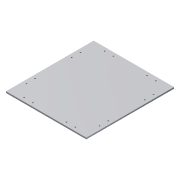
# Autodesk Inventor part: BackPlate
Saved by Autodesk Inventor 2014 (Build 180170000, 170)
## iProperties
Created: 2014-08-10
Part Number: BackPlate
Material: Generic
Document SubType Name: Modeling
Designer: Peele
Density: 1 g/cm^3
Appearance: White
Author: Peele
Autodesk Inventor part; units mm, degrees
ref_plane "YZ Plane" through (0, 0, 0) normal (1, 0, 0) x (0, 1, 0)
ref_plane "XZ Plane" through (0, 0, 0) normal (0, 1, 0) x (-1, 0, 0)
ref_plane "XY Plane" through (0, 0, 0) normal (0, 0, 1) x (1, 0, 0)
sketch "Sketch1" plane through (0, 0, 0) normal (0, 0, 1) x (1, 0, 0)
  line L0 (-112.5, -125) -> (112.5, -125)
  line L1 (112.5, -125) -> (112.5, 125)
  line L2 (112.5, 125) -> (-112.5, 125)
  line L3 (-112.5, 125) -> (-112.5, -125)
  line L4 (-112.5, -125) -> (112.5, 125) construction
  line L5 (112.5, -125) -> (-112.5, 125) construction
  point P0 (0, 0)
  dimension "d0" = 250
  dimension "d1" = 225
  constraints: 12 end point, 2 midpoint, 2 parallel, 1 horizontal, 1 perpendicular
  measures "d0" distance of L2.end L0.start
  measures "d1" distance of L1.end L2.end
extrude "Extrusion1" add sketch "Sketch1" along normal blind 5
sketch "Sketch2" plane through (0, 0, 5) normal (0, 0, 1) x (1, 0, 0)
  line L0 (112.5, -125) -> (112.5, 125) projected
  line L1 (112.5, 125) -> (-112.5, 125) projected
  line L2 (-112.5, 125) -> (-112.5, -125) projected
  circle A0 centre (-87.5, 137.5) radius 2.25
  circle A1 centre (-57.5, 137.5) radius 2.25
  circle A2 centre (57.5, 137.5) radius 2.25
  circle A3 centre (87.5, 137.5) radius 2.25
  circle A4 centre (125, 92.5) radius 2.25
  circle A5 centre (125, 62.5) radius 2.25
  circle A6 centre (-125, 92.5) radius 2.25
  circle A7 centre (-125, 62.5) radius 2.25
  line L3 (-112.5, 0) -> (-112.5, 125)
  line L4 (-112.5, 125) -> (112.5, 125)
  line L5 (112.5, 125) -> (112.5, 0)
  line L6 (112.5, 0) -> (137.5, 0)
  line L7 (137.5, 0) -> (137.5, 150)
  line L8 (137.5, 150) -> (-137.5, 150)
  line L9 (-137.5, 150) -> (-137.5, 0)
  line L10 (-137.5, 0) -> (-112.5, 0)
  point P0 (0, 0)
  dimension "d7" = 12.5
  dimension "d8" = 12.5
  dimension "d9" = 4.5
  dimension "d10" = 30
  dimension "d11" = 30
  dimension "d12" = 30
  dimension "d24" = 25
  dimension "d25" = 25
  dimension "d26" = 32.5
  dimension "d27" = 12.5
  dimension "d28" = 25
  dimension "d29" = 25
  constraints: 16 end point, 8 centre point, 7 equal radius, 5 horizontal alignment, 3 collinear, 3 perpendicular, 2 midpoint, 2 vertical alignment, 1 horizontal, 1 parallel
  measures "d7" distance from line of A0.centre L1
  measures "d8" distance from line of A6.centre L2
  measures "d9" diameter of A4
  measures "d10" distance of A3.centre A2.centre
  measures "d11" distance of A0.centre A1.centre
  measures "d12" distance of A5.centre A4.centre
  measures "d24" distance from line of A3.centre L0
  measures "d25" distance from line of A0.centre L2
  measures "d26" distance from line of A4.centre L1
  measures "d27" distance from line of A4.centre L0
  measures "d28" distance of L9.end L3.start
  measures "d29" distance between parallel lines of L8 L1
extrude "Extrusion2" add sketch "Sketch2" against normal blind 5
mirror "Mirror1" about plane through (0, 0, 0) normal (0, 1, 0) of "Extrusion2"
equation "\"d8\" = d7"
equation "\"d11\" = d10"
equation "\"d12\" = d10"
equation "\"d29\" = d28"
body "Solid1"
